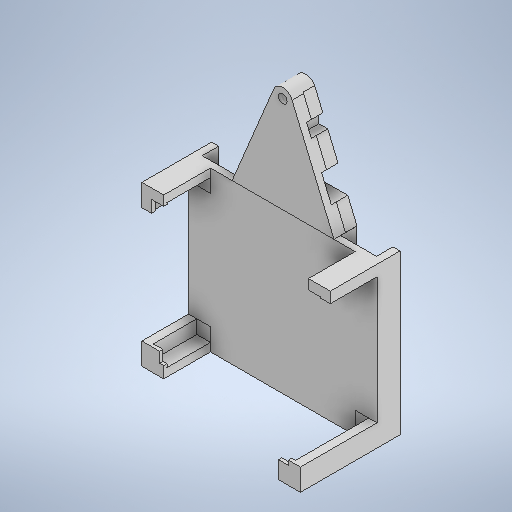
# Autodesk Inventor part: SENX_Mount
Saved by Autodesk Inventor 2025 (Build 290162010, 162A)
## iProperties
Created: 2024-06-25
Part Number: SENX_Mount
Material: Generic
Document SubType Name: Modeling
Designer: vncnt
Density: 1 g/cm^3
Appearance: Default
Author: vncnt
## iProperties of the stored document SEN5X_Mount_3DPrint.ipt
Created: 2024-06-27
Part Number: SEN5X_Mount_3DPrint
Material: Generic
Document SubType Name: Modeling
Designer: vncnt
Density: 1 g/cm^3
Appearance: Default
Author: vncnt
Autodesk Inventor part; units mm, degrees
note: some values were not read from the file. Chosen so that the rebuilt part matches the saved one: second side of "Extrusion3".
ref_plane "YZ Plane" through (0, 0, 0) normal (1, 0, 0) x (0, 1, 0)
sketch "Sketch1" plane through (0, 0, 0) normal (0, 0, 1) x (1, 0, 0)
  line L0 (26.15, 21.71) -> (26.15, -21.71)
  line L1 (-26.15, 21.71) -> (26.15, -21.71) construction
  line L2 (26.15, 21.71) -> (-26.15, -21.71) construction
  line L3 (28.65, -24.21) -> (28.65, 24.21)
  line L4 (-17.664706, 24.21) -> (11.881344, -16.283732) construction
  line L5 (22, 17) -> (-22, -17) construction
  line L6 (22, -24.21) -> (28.65, -24.21)
  line L7 (26.15, -21.71) -> (22, -21.71)
  line L8 (22, -21.71) -> (22, -24.21)
  line L9 (0, 21.71) -> (0, 40)
  line L10 (28.65, 24.21) -> (0, 24.21)
  line L11 (0, 21.71) -> (26.15, 21.71)
  line L12 (-26.15, 21.71) -> (-26.15, -21.71)
  line L13 (-28.65, -24.21) -> (-28.65, 24.21)
  line L14 (-22, -24.21) -> (-28.65, -24.21)
  line L15 (-26.15, -21.71) -> (-22, -21.71)
  line L16 (-22, -21.71) -> (-22, -24.21)
  line L17 (-28.65, 24.21) -> (0, 24.21)
  line L18 (0, 21.71) -> (-26.15, 21.71)
  line L19 (-22, -21.71) -> (22, -21.71)
  line L20 (22, -21.71) -> (22, -24.21)
  line L21 (22, -24.21) -> (-22, -24.21)
  line L22 (-22, -24.21) -> (-22, -21.71)
  point P0 (0, 0)
  point P1 (-11.881344, -16.283732)
  point P2 (-22, 17)
  dimension "d1" = 43.42
  dimension "d21" = 28.65
  dimension "d22" = 26.15
  constraints: 46 end point, 6 symmetric about line, 4 parallel, 3 midpoint, 3 perpendicular, 2 horizontal, 2 point on line, 1 vertical
  measures "d1" distance of L0.start L0.end
  measures "d21" distance between parallel lines of L3 L9
  measures "d22" distance of L9.start L0.start
extrude "Extrusion1" add sketch "Sketch1" along normal blind 22.3 contours L11 L9 L10 L3 L6 L8 L7 L0 | L18 L12 L15 L16 L14 L13 L17 L9 | L8 L21 L16 L19
sketch "Sketch4" plane through (-28.65, 24.21, 0) normal (0, 1, 0) x (1, 0, 0)
  line L0 (26.618, -3.5) -> (30.682, -3.5)
  line L1 (30.682, -3.5) -> (30.682, 3.5)
  line L2 (30.682, 3.5) -> (26.618, 3.5)
  line L3 (26.618, 3.5) -> (26.618, -3.5)
  line L4 (26.618, -3.5) -> (30.682, 3.5) construction
  line L5 (30.682, -3.5) -> (26.618, 3.5) construction
  line L6 (57.3, 0) -> (0, 0)
  line L7 (25.775621, 0) -> (33, 0)
  point P0 (28.65, 0)
  point P1 (26.618, 0)
  point P2 (30.682, 0)
  dimension "d23" = 4.064
  dimension "d24" = 7
  constraints: 14 end point, 2 midpoint, 2 parallel, 1 horizontal, 1 perpendicular, 1 point on line
  measures "d23" distance of L2.end L1.end
  measures "d24" distance of L1.end L0.end
extrude "Extrusion3" add sketch "Sketch4" along normal blind 31.75 contours L3 L2 L1 L6
sketch "Sketch6" plane through (28.65, -24.21, 0) normal (1, 0, 0) x (0, 0, -1)
  line L0 (-11.7, 45.12) -> (-2.3, 45.12)
  line L1 (-2.3, 45.12) -> (-2.3, 33.12)
  line L2 (-2.3, 33.12) -> (-11.7, 33.12)
  line L3 (-11.7, 33.12) -> (-11.7, 45.12)
  line L4 (-11.7, 45.12) -> (-2.3, 33.12) construction
  line L5 (-2.3, 45.12) -> (-11.7, 33.12) construction
  line L6 (0, 0) -> (0, 48.42) projected
  line L7 (0, 48.42) -> (-22.3, 48.42) projected
  point P0 (0, 24.21)
  point P1 (-7, 39.12)
  dimension "d38" = 9.4
  dimension "d39" = 12
  dimension "d40" = 2.3
  dimension "d41" = 3.3
  constraints: 12 end point, 2 midpoint, 2 parallel, 1 horizontal, 1 perpendicular
  measures "d38" distance of L1.end L2.end
  measures "d39" distance of L0.end L1.end
  measures "d40" distance between parallel lines of L6 L1
  measures "d41" distance between parallel lines of L7 L0
extrude "Extrusion4" cut sketch "Sketch6" against normal blind 20
sketch "Sketch8" plane through (2.032, 55.96, -3.5) normal (0, 0, -1) x (-1, 0, 0)
  line L0 (0, 0) -> (4.064, 0) projected
  line L1 (0, -31.75) -> (0, 0) projected
  point P0 (2.032, -55.96)
  point P1 (2.032, -2.5)
  point P2 (0, -80.17)
  dimension "d46" = 2.5
  dimension "d47" = 2.032
  measures "d46" distance from line of L0 point (2.032, -2.5)
  measures "d47" distance from line of L1 point (2.032, -2.5)
hole "Hole3" at (0, 53.46, -3.5) direction (0, 0, 1) diameter 2.6416 depth 10.979 thread size "6-32 UNC" class "2B" standard "ANSI Unified Screw Threads"
sketch "Sketch10" plane through (-28.65, -24.21, 22.3) normal (0, -1, 0) x (1, 0, 0)
  circle A0 centre (39, -11) radius 9.5
  line L0 (8.006, -5.4) -> (17.006, -5.4)
  line L1 (17.006, -5.4) -> (17.006, -20.4)
  line L2 (17.006, -20.4) -> (8.006, -20.4)
  line L3 (8.006, -20.4) -> (8.006, -5.4)
  line L4 (57.3, -22.3) -> (57.3, 0) projected
  line L5 (0, -22.3) -> (57.3, -22.3) projected
  line L6 (0, -22.3) -> (57.3, -22.3) projected
  point P0 (28.65, -22.3)
  point P1 (30.682, -22.3)
  point P2 (28.65, -22.3)
  point P3 (26.618, -22.3)
  dimension "d59" = 18.3
  dimension "d60" = 11.3
  dimension "d61" = 19
  dimension "d62" = 9
  dimension "d63" = 15
  dimension "d64" = 40.294
  dimension "d65" = 1.9
  constraints: 8 end point, 2 parallel, 1 centre point, 1 horizontal, 1 midpoint, 1 perpendicular
  measures "d59" distance from line of L4 A0.centre
  measures "d60" vertical distance of point (28.65, -22.3) A0.centre
  measures "d61" diameter of A0
  measures "d62" distance of L1.end L2.end
  measures "d63" distance of L0.end L1.end
  measures "d64" distance between parallel lines of L4 L1
  measures "d65" distance between parallel lines of L6 L2
extrude "Extrusion7" cut sketch "Sketch10" against normal blind 31.75
sketch "Sketch12" plane through (28.65, 24.21, 22.3) normal (0, 1, 0) x (1, 0, 0)
  line L0 (-2.5, 22.3) -> (-54.8, 22.3)
  line L1 (-16.2, 22.3) -> (-17, 22.3)
  line L2 (-54.8, 22.3) -> (-2.5, 22.3)
  line L3 (-41, 22.3) -> (-46.57683, 22.3)
  line L4 (-48, 22.3) -> (-39.837, 22.3)
  line L5 (-17.463, 22.3) -> (-9.463, 22.3)
  line L6 (-30.682, 25.8) -> (-30.682, 22.3)
  line L7 (-26.618, 22.3) -> (-26.618, 25.8)
  line L8 (0, 22.3) -> (-57.3, 22.3)
  line L9 (-57.3, 22.3) -> (0, 22.3)
  line L10 (0, 22.3) -> (0, 29.3)
  line L11 (0, 29.3) -> (-57.3, 29.3)
  line L12 (-57.3, 29.3) -> (-57.3, 22.3)
  line L13 (-28.65, 27.8) -> (-28.65, 30.382901)
  line L14 (-5.155, 29.3) -> (-10.235, 29.3)
  line L15 (-10.235, 29.3) -> (-10.235, 23)
  line L16 (-5.155, 23) -> (-5.155, 29.3)
  line L17 (-20.395, 29.3) -> (-25.475, 29.3)
  line L18 (-25.475, 29.3) -> (-25.475, 19.5)
  line L19 (-20.395, 23) -> (-20.395, 29.3)
  line L20 (-31.825, 29.3) -> (-36.905, 29.3)
  line L21 (-36.905, 29.3) -> (-36.905, 23)
  line L22 (-31.825, 19.5) -> (-31.825, 29.3)
  line L23 (-47.065, 29.3) -> (-52.145, 29.3)
  line L24 (-52.145, 29.3) -> (-52.145, 23)
  line L25 (-47.065, 19.5) -> (-47.065, 29.3)
  line L26 (-55.145, 22.3) -> (-55.145, 29.3)
  line L27 (-44.065, 29.3) -> (-44.065, 22.3)
  line L28 (-39.905, 22.3) -> (-39.905, 29.3)
  line L29 (-28.825, 29.3) -> (-28.825, 22.3)
  line L30 (-28.475, 22.3) -> (-28.475, 29.3)
  line L31 (-27.475, 27.8) -> (-26.618, 27.8)
  line L32 (-17.395, 29.3) -> (-17.395, 22.3)
  line L33 (-13.235, 22.3) -> (-13.235, 29.3)
  line L34 (-2.155, 29.3) -> (-2.155, 22.3)
  line L35 (-57.3, 22.3) -> (0, 22.3)
  line L36 (0, 24.3) -> (-57.3, 24.3)
  point P0 (-28.65, 22.3)
  point P1 (-30.682, 22.3)
  point P2 (-28.65, 28.09145)
  point P3 (-25.475, 24.4)
  point P4 (-31.825, 24.4)
  point P5 (-47.065, 24.4)
  point P6 (-2.155, 24.3)
  point P7 (-13.235, 24.3)
  point P8 (-17.395, 24.3)
  point P9 (-26.618, 24.3)
  point P10 (-30.682, 24.3)
  point P11 (-39.905, 24.3)
  point P12 (-44.065, 24.3)
  point P13 (-55.145, 24.3)
  point P14 (-28.475, 24.3)
  point P15 (-28.825, 24.3)
  dimension "d85" = 7
  dimension "d258" = 23.495
  dimension "d259" = 18.415
  dimension "d260" = 8.255
  dimension "d261" = 3.175
  dimension "d262" = 3.175
  dimension "d263" = 2.032
  dimension "d264" = 2.032
  dimension "d265" = 4.064
  dimension "d266" = 8.255
  dimension "d267" = 18.415
  dimension "d268" = 23.495
  dimension "d269" = 3
  dimension "d270" = 3
  dimension "d271" = 3
  dimension "d272" = 3
  dimension "d273" = 11.08
  dimension "d274" = 5
  dimension "d284" = 3
  dimension "d285" = 3
  dimension "d286" = 3
  dimension "d287" = 3
  constraints: 62 end point, 17 point on line, 9 horizontal, 9 parallel, 7 perpendicular, 3 midpoint, 1 collinear, 1 vertical, 15 other
  measures "d258" distance from line of L16 point (-28.65, 28.091)
  measures "d259" distance between parallel lines of L15 L13
  measures "d260" distance between parallel lines of L13 L19
  measures "d261" distance from line of L13 point (-25.475, 24.4)
  measures "d262" distance from line of L13 point (-31.825, 24.4)
  measures "d263" distance between parallel lines of L7 L13
  measures "d264" distance between parallel lines of L13 L6
  measures "d265" distance between parallel lines of L7 L6
  measures "d266" distance between parallel lines of L21 L13
  measures "d267" distance from line of L13 point (-47.065, 24.4)
  measures "d268" distance between parallel lines of L13 L24
  measures "d269" distance between parallel lines of L24 L26
  measures "d270" distance between parallel lines of L21 L28
  measures "d271" distance between parallel lines of L18 L30
  measures "d272" distance between parallel lines of L15 L33
  measures "d273" distance between parallel lines of L34 L33
  measures "d284" distance between parallel lines of L27 L25
  measures "d285" distance between parallel lines of L22 L29
  measures "d286" distance between parallel lines of L19 L32
  measures "d287" distance between parallel lines of L16 L34
extrude "Extrusion8" add sketch "Sketch12" against normal up to surface (48.42 mm away) contours L0 L33 L36 L34 L8 | L34 L36 L10 L8 | L0 L32 L36 L33 | L34 L11 L10 L36 | L36 L32 L11 L33 | L32 L0 L18 L36 | L18 L0 L7 L36 | L7 L0 L30 L36 | L30 L36 L29 L11 | L30 L0 L29 L36 | L29 L0 L6 L36 | L6 L0 L22 L36 | L22 L0 L28 L36 | L28 L36 L27 L11 | L28 L0 L27 L36 | L27 L0 L25 L36 | L25 L0 L8 L26 L36 | L26 L36 L12 L11 | L26 L8 L12 L36
sketch "Sketch16" plane through (2.032, 24.21, 0) normal (0, 1, 0) x (1, 0, 0)
  line L0 (0, 3.5) -> (15.560994, 3.5)
  line L1 (24.118, 0) -> (-28.182, 0)
  line L2 (0, 3.5) -> (15.560994, 3.5)
  line L3 (15.560994, 3.5) -> (15.560994, 0)
  line L4 (15.560994, 0) -> (0, 0)
  line L5 (0, 0) -> (0, 3.5)
  line L6 (0, 3.5) -> (0, 0)
  constraints: 10 end point, 2 horizontal, 1 parallel, 1 perpendicular, 1 point on line, 1 vertical
extrude "Extrusion12" add sketch "Sketch16" along normal up to surface (31.75 mm away)
sketch "Sketch18" plane through (-28.65, 55.96, 0) normal (0, 1, 0) x (1, 0, 0)
  line L0 (26.618, 3.5) -> (46.242994, 3.5)
  line L1 (26.618, 3.5) -> (46.242994, 3.5)
  line L2 (46.242994, 3.5) -> (46.242994, 0)
  line L3 (46.242994, 0) -> (26.618, 0)
  line L4 (26.618, 0) -> (26.618, 3.5)
  point P0 (28.65, 0)
  point P1 (30.682, 3.5)
  point P2 (30.682, 3.5)
  constraints: 8 end point, 2 parallel, 1 horizontal, 1 perpendicular
extrude "Extrusion14" add sketch "Sketch18" along normal blind 3
sketch "Sketch19" plane through (-2.032, 24.21, -3.5) normal (-1, 0, 0) x (0, 0, 1)
  line L0 (0, 34.75) -> (3.5, 34.75)
  line L1 (3.5, 34.75) -> (3.5, 0)
  line L2 (3.5, 0) -> (0, 0)
  line L3 (0, 0) -> (0, 34.75)
  constraints: 8 end point, 2 parallel, 1 horizontal, 1 perpendicular
extrude "Extrusion15" add sketch "Sketch19" along normal up to surface (13.383 mm away)
sketch "Sketch21" plane through (0, 0, 22.3) normal (0, 0, 1) x (1, 0, 0)
  line L0 (-38, 31) -> (34, 31)
  line L1 (34, 31) -> (34, -30)
  line L2 (34, -30) -> (-38, -30)
  line L3 (-38, -30) -> (-38, 31)
  line L4 (34, -30) -> (12, -30)
  line L5 (12, -30) -> (12, -12)
  line L6 (12, -12) -> (34, -12)
  line L7 (34, -12) -> (34, -30)
  point P0 (0, 0)
  constraints: 16 end point, 4 parallel, 2 horizontal, 2 perpendicular
extrude "Extrusion17" cut sketch "Sketch21" against normal blind 9.0932 contours L0 L1 L6 L5 L2 L3
sketch "Sketch22" plane through (0, 0, 22.3) normal (0, 0, 1) x (1, 0, 0)
  line L0 (28.65, 24.21) -> (28.65, -24.21)
  line L1 (26.15, 21.71) -> (26.15, -21.71)
  line L2 (28.65, -24.21) -> (26.15, -24.21)
  line L3 (28.65, -17.56) -> (28.65, -24.21)
  line L4 (22, -21.709086) -> (22, -21.559086)
  line L5 (26, -21.709086) -> (26, -21.71)
  line L6 (26, -17.56) -> (22, -17.56)
  line L7 (22, -17.56) -> (22, -21.559086)
  line L8 (22, -17.56) -> (25.250206, -17.56)
  line L9 (22, -18.943211) -> (22, -17.56)
  line L10 (22, -17.56) -> (28.65, -17.56)
  line L11 (28.65, -17.56) -> (28.65, -24.21)
  line L12 (28.65, -24.21) -> (22, -24.21)
  line L13 (22, -24.21) -> (22, -17.56)
  line L14 (22, -17.56) -> (25, -17.56)
  line L15 (25, -17.56) -> (25, -18.937917)
  line L16 (25, -18.937917) -> (22, -18.937917)
  line L17 (22, -18.937917) -> (22, -17.56)
  point P0 (0, 0)
  constraints: 32 end point, 5 horizontal, 5 parallel, 3 perpendicular
extrude "Extrusion18" add sketch "Sketch22" along normal blind 1 contours L0 L2 L12 L13 L4 L7 L16 L15 L6 L10
sketch "Sketch23" plane through (0, 0, 13.2068) normal (0, 0, 1) x (1, 0, 0)
  line L0 (-28.65, -21.71) -> (-28.65, -24.216707)
  line L1 (-28.65, -24.216707) -> (-22, -24.216707)
  line L2 (-26.15, -17.56) -> (-26, -17.56)
  line L3 (-26, -17.56) -> (-23.25, -17.56)
  line L4 (-23.25, -17.56) -> (-23.25, -20.707959)
  line L5 (-23.25, -17.56) -> (-28.65, -17.56)
  line L6 (-28.65, -17.56) -> (-28.65, -24.216707)
  line L7 (-28.65, -24.216707) -> (-23.25, -24.216707)
  line L8 (-23.25, -20.707959) -> (-23.25, -17.56)
  line L9 (-22, -24.216707) -> (-28.65, -24.216707)
  line L10 (-28.65, -24.216707) -> (-28.65, -21.71)
  line L11 (-23.25, -20.707959) -> (-22, -20.707959)
  line L12 (-22, -20.707959) -> (-22, -24.216707)
  point P0 (0, 0)
  point P1 (-26.15, -21.71)
  constraints: 26 end point, 4 horizontal, 4 parallel, 3 perpendicular
extrude "Extrusion19" add sketch "Sketch23" along normal blind 1
ref_plane "Work Plane3" through (-9.255, -24.21, -3.5) normal (0, 0, -1) x (-1, 0, 0)
sketch "Sketch26" plane through (-9.255, -24.21, -3.5) normal (0, 0, -1) x (-1, 0, 0)
  circle A0 centre (-9.255, 77.67) radius 1.3208
  circle A1 centre (-4.81, 76.4) radius 1.75
  circle A2 centre (-12.43, 58.62) radius 3.5
  circle A3 centre (-2.3208, 56.588) radius 3.5
  circle A4 centre (-9.255, 77.67) radius 1.3208
  circle A5 centre (-14.97, 71.32) radius 1.75
  circle A6 centre (-2.27, 68.78) radius 1.75
  line L0 (-4.02, 67.03) -> (-0.52, 67.03)
  line L1 (-0.52, 70.53) -> (-4.02, 70.53)
  line L2 (-4.02, 70.53) -> (-4.02, 67.03)
  line L3 (-6.56, 74.65) -> (-3.06, 74.65)
  line L4 (-3.06, 74.65) -> (-3.06, 78.15)
  line L5 (-6.56, 78.15) -> (-6.56, 74.65)
  line L6 (-16.72, 69.57) -> (-13.22, 69.57)
  line L7 (-13.22, 69.57) -> (-13.22, 73.07)
  line L8 (-13.22, 73.07) -> (-16.72, 73.07)
  line L9 (-16.72, 73.07) -> (-26.212994, 73.07)
  line L10 (-26.212994, 73.07) -> (-26.212994, 69.57)
  line L11 (-26.212994, 69.57) -> (-16.72, 69.57)
  line L12 (-0.52, 70.53) -> (7.157192, 70.53)
  line L13 (7.157192, 70.53) -> (7.157192, 67.03)
  line L14 (7.157192, 67.03) -> (-0.52, 67.03)
  line L15 (-3.06, 81.95) -> (-3.06, 78.15)
  line L16 (-5.8208, 60.088) -> (1.1792, 60.088)
  line L17 (1.1792, 53.088) -> (-5.8208, 53.088)
  line L18 (-5.8208, 53.088) -> (-5.8208, 60.088)
  line L19 (-15.93, 55.12) -> (-8.93, 55.12)
  line L20 (-8.93, 55.12) -> (-8.93, 62.12)
  line L21 (-8.93, 62.12) -> (-15.93, 62.12)
  line L22 (1.1792, 60.088) -> (7.189214, 60.088)
  line L23 (7.189214, 60.088) -> (7.189214, 53.088)
  line L24 (7.189214, 53.088) -> (1.1792, 53.088)
  line L25 (-15.93, 62.12) -> (-26.847994, 62.12)
  line L26 (-26.847994, 62.12) -> (-26.847994, 55.12)
  line L27 (-26.847994, 55.12) -> (-15.93, 55.12)
  line L28 (-3.06, 74.65) -> (-6.56, 74.65)
  line L29 (-6.56, 74.65) -> (-6.56, 81.95)
  line L30 (-6.56, 81.95) -> (-3.06, 81.95)
  line L31 (-3.06, 81.95) -> (-3.06, 74.65)
  line L32 (-26.212994, 73.07) -> (-13.22, 73.07)
  line L33 (-13.22, 73.07) -> (-13.22, 69.57)
  line L34 (-13.22, 69.57) -> (-26.212994, 69.57)
  line L35 (-26.212994, 69.57) -> (-26.212994, 73.07)
  line L36 (-26.847994, 62.12) -> (-8.93, 62.12)
  line L37 (-8.93, 62.12) -> (-8.93, 55.12)
  line L38 (-8.93, 55.12) -> (-26.847994, 55.12)
  line L39 (-26.847994, 55.12) -> (-26.847994, 62.12)
  line L40 (-5.8208, 60.088) -> (7.189214, 60.088)
  line L41 (7.189214, 60.088) -> (7.189214, 53.088)
  line L42 (7.189214, 53.088) -> (-5.8208, 53.088)
  line L43 (-5.8208, 53.088) -> (-5.8208, 60.088)
  line L44 (-4.02, 70.53) -> (7.157192, 70.53)
  line L45 (7.157192, 70.53) -> (7.157192, 67.03)
  line L46 (7.157192, 67.03) -> (-4.02, 67.03)
  line L47 (-4.02, 67.03) -> (-4.02, 70.53)
  point P0 (-28.83917, 91.985835)
  point P1 (-17.13917, 89.985835)
  point P2 (-14.59917, 99.605835)
  point P3 (-15.09917, 100.105835)
  point P4 (-29.709534, 90.493427)
  point P5 (-17.63917, 89.485412)
  point P6 (-29.709534, 91.478243)
  point P7 (-17.63917, 89.485412)
  point P8 (-17.63917, 89.985835)
  point P9 (-17.63917, 91.986116)
  point P10 (-3.20917, 100.105835)
  point P11 (-0.66917, 89.485412)
  point P12 (-2.27, 70.53)
  point P13 (-2.27, 67.03)
  point P14 (-4.02, 68.78)
  point P15 (1.1792, 53.088)
  point P16 (-2.3208, 60.088)
  point P17 (-2.3208, 53.088)
  point P18 (-12.43, 55.12)
  point P19 (-12.43, 62.12)
  point P20 (-5.8208, 56.588)
  point P21 (-6.56, 78.15)
  point P22 (-8.93, 58.62)
  dimension "d225" = 3.5
  dimension "d230" = 7
  dimension "d231" = 7
  dimension "d240" = 3.5
  dimension "d242" = 5.715
  dimension "d243" = 6.35
  dimension "d244" = 6.985
  dimension "d245" = 8.89
  dimension "d246" = 4.445
  dimension "d247" = 1.27
  dimension "d248" = 3.5
  dimension "d249" = 3.175
  dimension "d250" = 19.05
  dimension "d251" = 6.9342
  dimension "d252" = 21.082
  dimension "d253" = 7
  constraints: 96 end point, 19 parallel, 14 horizontal, 12 perpendicular, 7 centre point, 1 concentric
  measures "d225" diameter of A5
  measures "d230" diameter of A2
  measures "d231" diameter of A3
  measures "d240" diameter of A6
  measures "d242" horizontal distance of A5.centre A0.centre
  measures "d243" vertical distance of A5.centre A0.centre
  measures "d244" horizontal distance of A6.centre A0.centre
  measures "d245" vertical distance of A0.centre A6.centre
  measures "d246" horizontal distance of A1.centre A0.centre
  measures "d247" vertical distance of A0.centre A1.centre
  measures "d248" diameter of A1
  measures "d249" horizontal distance of A2.centre A0.centre
  measures "d250" vertical distance of A2.centre A0.centre
  measures "d251" horizontal distance of A3.centre A0.centre
  measures "d252" vertical distance of A0.centre A3.centre
  measures "d253" distance of L21.end L20.end
extrude "Extrusion22" cut sketch "Sketch26" against normal up to surface (1.5 mm away) contours A1 | L4 L3 A1 | A1 L5 L29 L30 L15 L4 | A1 L3 L5 | A2 | L20 L19 A2 | A2 L21 L20 | A2 L19 L27 L26 L25 L21 | A3 | A3 L16 L22 L23 L24 L17 | A3 L18 L16 | L17 L18 A3 | A5 | L7 L6 A5 | A5 L8 L7 | A5 L6 L11 L10 L9 L8 | A6 | A6 L1 L12 L13 L14 L0 | A6 L2 L1 | L0 L2 A6
ref_plane "Work Plane2" through (17.565, -24.21, -3.5) normal (0, 0, -1) x (-1, 0, 0)
sketch "Sketch27" plane through (17.565, -24.21, -3.5) normal (0, 0, -1) x (-1, 0, 0)
  circle A0 centre (17.565, 77.67) radius 1.3208
  circle A1 centre (17.565, 77.67) radius 3
  line L0 (32.98, 48.42) -> (44.06, 48.42)
  line L1 (-0.027994, 83.17) -> (32.98, 83.17)
  line L2 (32.98, 83.17) -> (32.98, 48.42)
  line L3 (32.98, 48.42) -> (-0.027994, 48.42)
  line L4 (-0.027994, 48.42) -> (-0.027994, 83.17)
  line L5 (2, 48.42) -> (14.868236, 78.98433)
  line L6 (32.98, 48.42) -> (20.334958, 78.822099)
  point P0 (14.740252, 78.680345)
  dimension "d275" = 6
  constraints: 12 end point, 3 point on circle, 2 parallel, 1 centre point, 1 coincident, 1 horizontal, 1 perpendicular, 1 point on line, 1 tangent
  measures "d275" diameter of A1
sketch "Sketch27 outline for Extrusion23" plane through (17.565, -24.21, -3.5) normal (0, 0, -1) x (-1, 0, 0)
  line L0 (32.98, 48.42) -> (32.98, 83.17)
  line L1 (20.334958, 78.822099) -> (32.98, 48.42)
  arc A0 (14.740252, 78.680345) -> (20.334958, 78.822099) centre (17.565, 77.67) cw
  line L2 (2, 48.42) -> (14.740252, 78.680345)
  line L3 (-0.027994, 48.42) -> (2, 48.42)
  line L4 (-0.027994, 83.17) -> (-0.027994, 48.42)
  line L5 (32.98, 83.17) -> (-0.027994, 83.17)
extrude "Extrusion23" cut sketch "Sketch27 outline for Extrusion23" against normal through all
sketch "Sketch28" plane through (0, 0, 13.2068) normal (0, 0, 1) x (1, 0, 0)
  line L0 (-15.415, -24.21) -> (-26.495, -24.21)
  line L1 (26.495, 24.21) -> (15.415, 24.21)
  line L2 (-22, -24.21) -> (22, -24.21)
  line L3 (22, 24.21) -> (-22, 24.21)
  line L4 (-22, 17.56) -> (-28.65, 17.56)
  line L5 (28.65, -17.56) -> (22, -17.56)
  line L6 (22, 20.91) -> (28.65, 20.91)
  line L7 (28.65, 8.91) -> (28.65, 20.91)
  line L8 (28.65, 20.91) -> (28.65, -17.56)
  line L9 (22, -24.21) -> (22, -17.56)
  line L10 (22, 20.91) -> (22, 24.21)
  line L11 (-22, 24.21) -> (-22, 17.56)
  line L12 (-22, -17.56) -> (-22, -24.21)
  line L13 (26.495, 24.21) -> (26.495, -24.21)
  line L14 (22, -17.56) -> (26.495, -17.56)
  line L15 (26.495, -17.56) -> (26.495, -20.638483)
  line L16 (22, -20.638483) -> (22, -17.56)
  line L17 (-28.65, 17.56) -> (-28.65, -17.56)
  line L18 (-28.65, -17.56) -> (-22, -17.56)
  line L19 (-23.25, -17.56) -> (-26.15, -17.56)
  point P0 (0, 0)
  point P1 (17.592994, 24.21)
  point P2 (17.592994, 24.21)
  point P3 (26.495, 20.91)
  dimension "d277" = 6.65
  constraints: 30 end point, 6 parallel, 4 perpendicular, 4 point on line, 3 horizontal, 1 collinear, 1 vertical
  measures "d277" distance between parallel lines of L3 L4
extrude "Extrusion24" cut sketch "Sketch28" along normal blind 11 and the other way blind 13.207 contours L0 L12 L18 L17 L4 L11 L3 L1 L10 L6 L13 L5 L9 L2 | L13 L6 L7 L8 L5
sketch "Sketch29" plane through (11.255, 24.21, -3.5) normal (0, 0, -1) x (-1, 0, 0)
  line L0 (26.67, 0) -> (-4.31, 0)
  line L1 (-4.31, 0) -> (26.67, 0)
  circle A0 centre (11.255, 29.25) radius 1.3208
  arc A1 (14.024958, 30.402099) -> (8.427859, 30.25363) centre (11.255, 29.25) ccw
  line L2 (26.67, 0) -> (-4.31, 0)
  line L3 (1.457993, 13.7) -> (11.58, 13.7)
  line L4 (11.58, 13.7) -> (1.458189, 13.7)
  line L5 (11.58, 13.7) -> (11.58, 6.7)
  line L6 (11.58, 13.7) -> (11.58, 6.7)
  line L7 (11.58, 6.7) -> (-1.489061, 6.7)
  line L8 (14.6892, 11.668) -> (21.816968, 11.668)
  line L9 (14.6892, 11.668) -> (21.816968, 11.668)
  line L10 (14.6892, 4.668) -> (14.6892, 11.668)
  line L11 (14.6892, 11.668) -> (14.6892, 4.668)
  line L12 (14.6892, 4.668) -> (24.728455, 4.668)
  line L13 (16.49, 18.61) -> (16.49, 22.11)
  line L14 (16.49, 22.11) -> (16.49, 18.61)
  line L15 (16.49, 18.61) -> (18.929606, 18.61)
  line L16 (16.49, 22.11) -> (17.473863, 22.11)
  line L17 (13.95, 26.23) -> (13.95, 30.567943)
  line L18 (13.95, 26.23) -> (15.760245, 26.23)
  line L19 (13.95, 26.23) -> (13.95, 30.567943)
  line L20 (6.068177, 24.65) -> (7.29, 24.65)
  line L21 (6.068177, 24.65) -> (7.29, 24.65)
  line L22 (7.29, 24.65) -> (7.29, 21.15)
  line L23 (7.29, 24.65) -> (7.29, 21.15)
  line L24 (7.29, 21.15) -> (4.594905, 21.15)
  line L25 (26.67, 0) -> (24.728455, 4.668)
  line L26 (21.816968, 11.668) -> (18.929606, 18.61)
  line L27 (17.473863, 22.11) -> (15.760245, 26.23)
  line L28 (-1.489061, 6.7) -> (-4.31, 0)
  line L29 (8.561399, 30.5708) -> (6.068531, 24.65)
  line L30 (4.594905, 21.15) -> (1.458189, 13.7)
  point P0 (11.255, -24.21)
  point P1 (6.068531, 24.65)
  point P2 (1.458189, 13.7)
  constraints: 45 end point, 6 collinear, 5 perpendicular, 4 point on circle, 3 tangent, 3 vertical, 2 horizontal, 2 point on line, 1 centre point, 1 coincident
extrude "Extrusion25" add sketch "Sketch29" along normal up to surface (3.5 mm away) contours L0 L28 L7 L5 L3 L30 L24 L22 L20 L29 A1 L17 L18 L27 L16 L13 L15 L26 L8 L10 L12 L25
sketch "Sketch30" plane through (0, 0, 13.2068) normal (0, 0, 1) x (1, 0, 0)
  line L0 (-26.15, 17.56) -> (-26.15, 21.71)
  line L1 (-22, 24.21) -> (-26.15, 24.21)
  line L2 (-26.15, 21.71) -> (-22, 21.71)
  line L3 (-22, 21.71) -> (-22, 24.21)
  line L4 (-28.65, 17.56) -> (-22, 17.56)
  line L5 (-26.15, 24.21) -> (-28.65, 24.21)
  line L6 (-28.65, 24.21) -> (-28.65, 17.56)
  line L7 (-28.65, 17.56) -> (-26.15, 17.56)
  line L8 (-26.15, 17.56) -> (-26.15, 21.71)
  line L9 (22, 24.21) -> (22, 21.71)
  line L10 (22, 24.21) -> (28.65, 24.21)
  line L11 (22, 21.71) -> (22, 24.21)
  line L12 (26.15, 20.91) -> (28.65, 20.91)
  line L13 (26.15, 20.91) -> (28.65, 20.91)
  line L14 (26.15, 21.71) -> (26.15, 20.91)
  line L15 (28.65, 24.21) -> (28.65, 20.91)
  line L16 (26.15, 21.71) -> (22, 21.71)
  line L17 (-22, 17.56) -> (-25.65, 17.56)
  line L18 (-25.65, 17.56) -> (-25.65, 21.21)
  line L19 (-25.65, 21.21) -> (-22, 21.21)
  line L20 (-22, 21.21) -> (-22, 17.56)
  line L21 (-22, 22) -> (-22, 20.91)
  line L22 (-26.645103, 17.56) -> (-23.469692, 17.56)
  line L23 (21.056081, 19.9) -> (25.65, 19.9)
  line L24 (25.65, 19.9) -> (25.65, 21.21)
  line L25 (25.65, 21.21) -> (21.056081, 21.21)
  line L26 (21.056081, 21.21) -> (21.056081, 19.9)
  line L27 (22, 24.21) -> (22, 20.91)
  line L28 (22, 21.71) -> (22, 20.91)
  line L29 (22, 20.91) -> (27, 20.91)
  point P0 (0, 0)
  point P1 (-23.825, 21.21)
  point P2 (23.353041, 21.21)
  point P3 (25.65, 20.91)
  point P4 (22, 21.21)
  dimension "d291" = 0.5
  dimension "d292" = 0.5
  dimension "d293" = 0.5
  dimension "d294" = 0.5
  constraints: 50 end point, 8 parallel, 7 point on line, 6 horizontal, 3 perpendicular, 2 midpoint, 1 collinear, 1 vertical
  measures "d291" distance from line of L2 point (-23.825, 21.21)
  measures "d292" distance between parallel lines of L0 L18
  measures "d293" distance from line of L16 point (23.353, 21.21)
  measures "d294" distance between parallel lines of L14 L24
extrude "Extrusion26" add sketch "Sketch30" along normal blind 1 contours L4 L6 L5 L1 L3 L2 L0 | L0 L2 L21 L19 L18 L4 | L10 L15 L12 L14 L16 L9 | L16 L14 L29 L24 L25 L27
body "Solid1"
